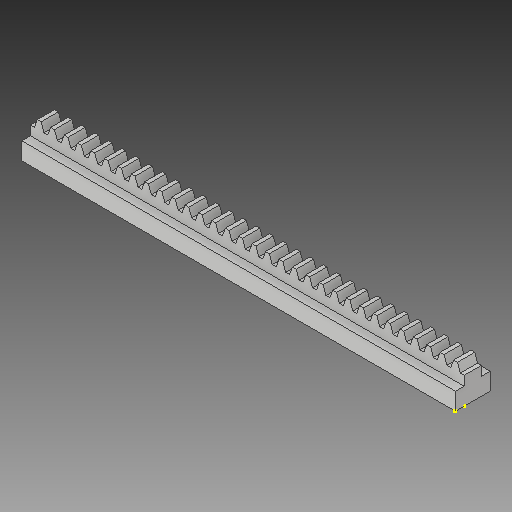
# Autodesk Inventor part: cremallera
Saved by Autodesk Inventor 2018.2 (Build 222227000, 227)
## iProperties
Created: 2016-05-04
Part Number: cremallera
Material: Genérico
Document SubType Name: Modeling
Designer: Usuario
Density: 1 g/cm^3
Appearance: Valor por defecto
Author: Usuario
Autodesk Inventor part; units mm, degrees
ref_plane "YZ Plane" through (0, 0, 0) normal (1, 0, 0) x (0, 1, 0)
ref_plane "XZ Plane" through (0, 0, 0) normal (0, 1, 0) x (-1, 0, 0)
ref_plane "XY Plane" through (0, 0, 0) normal (0, 0, 1) x (1, 0, 0)
sketch "Boceto1" plane through (0, 0, 0) normal (1, 0, 0) x (0, 1, 0)
  point P0 (0, 0)
extrude "Extrusión1" [suppressed]
sketch "Boceto2" plane through (0, 0, 0) normal (0, 0, 1) x (1, 0, 0)
  point P0 (0, 0)
sketch "Boceto3" plane through (0, 10, -5) normal (0, 0, 1) x (1, 0, 0)
  line L0 (227.2104, 2.6715) -> (229.8777, 10)
  line L1 (233.3764, 10) -> (236.0437, 2.6715)
  line L2 (214.787, 2.6715) -> (217.4544, 10)
  line L3 (220.953, 10) -> (223.6204, 2.6715)
  line L4 (202.3637, 2.6715) -> (205.031, 10)
  line L5 (208.5297, 10) -> (211.197, 2.6715)
  line L6 (189.9403, 2.6715) -> (192.6077, 10)
  line L7 (196.1063, 10) -> (198.7737, 2.6715)
  line L8 (177.517, 2.6715) -> (180.1843, 10)
  line L9 (183.683, 10) -> (186.3503, 2.6715)
  line L10 (165.0936, 2.6715) -> (167.761, 10)
  line L11 (171.2596, 10) -> (173.927, 2.6715)
  line L12 (152.6702, 2.6715) -> (155.3376, 10)
  line L13 (158.8362, 10) -> (161.5036, 2.6715)
  line L14 (140.2469, 2.6715) -> (142.9143, 10)
  line L15 (146.4129, 10) -> (149.0803, 2.6715)
  line L16 (127.8235, 2.6715) -> (130.4909, 10)
  line L17 (133.9895, 10) -> (136.6569, 2.6715)
  line L18 (115.4002, 2.6715) -> (118.0675, 10)
  line L19 (121.5662, 10) -> (124.2335, 2.6715)
  line L20 (102.9768, 2.6715) -> (105.6442, 10)
  line L21 (109.1428, 10) -> (111.8102, 2.6715)
  line L22 (90.5535, 2.6715) -> (93.2208, 10)
  line L23 (96.7195, 10) -> (99.3868, 2.6715)
  line L24 (78.1301, 2.6715) -> (80.7975, 10)
  line L25 (84.2961, 10) -> (86.9635, 2.6715)
  line L26 (65.7067, 2.6715) -> (68.3741, 10)
  line L27 (71.8728, 10) -> (74.5401, 2.6715)
  line L28 (53.2834, 2.6715) -> (55.9508, 10)
  line L29 (59.4494, 10) -> (62.1168, 2.6715)
  line L30 (40.86, 2.6715) -> (43.5274, 10)
  line L31 (47.0261, 10) -> (49.6934, 2.6715)
  line L32 (28.4367, 2.6715) -> (31.104, 10)
  line L33 (34.6027, 10) -> (37.2701, 2.6715)
  line L34 (16.0133, 2.6715) -> (18.6807, 10)
  line L35 (22.1793, 10) -> (24.8467, 2.6715)
  line L36 (3.59, 2.6715) -> (6.2573, 10)
  line L37 (9.756, 10) -> (12.4234, 2.6715)
  line L38 (239.6337, 2.6715) -> (242.3011, 10)
  line L39 (245.7997, 10) -> (248.4671, 2.6715)
  line L40 (248.4671, 2.6715) -> (250, 2.6715)
  line L41 (0, 0) -> (250, 0) projected
  line L42 (3.59, 2.6715) -> (0, 2.6715)
  line L43 (0, 0) -> (0, 10) projected
  line L44 (0, 2.6715) -> (0, 10)
  line L45 (0, 10) -> (6.2573, 10)
  line L46 (9.756, 10) -> (18.6807, 10)
  line L47 (12.4234, 2.6715) -> (16.0133, 2.6715)
  line L48 (236.0437, 2.6715) -> (239.6337, 2.6715)
  line L49 (223.6204, 2.6715) -> (227.2104, 2.6715)
  line L50 (211.197, 2.6715) -> (214.787, 2.6715)
  line L51 (198.7737, 2.6715) -> (202.3637, 2.6715)
  line L52 (186.3503, 2.6715) -> (189.9403, 2.6715)
  line L53 (173.927, 2.6715) -> (177.517, 2.6715)
  line L54 (161.5036, 2.6715) -> (165.0936, 2.6715)
  line L55 (149.0803, 2.6715) -> (152.6702, 2.6715)
  line L56 (136.6569, 2.6715) -> (140.2469, 2.6715)
  line L57 (124.2335, 2.6715) -> (127.8235, 2.6715)
  line L58 (111.8102, 2.6715) -> (115.4002, 2.6715)
  line L59 (99.3868, 2.6715) -> (102.9768, 2.6715)
  line L60 (86.9635, 2.6715) -> (90.5535, 2.6715)
  line L61 (74.5401, 2.6715) -> (78.1301, 2.6715)
  line L62 (62.1168, 2.6715) -> (65.7067, 2.6715)
  line L63 (49.6934, 2.6715) -> (53.2834, 2.6715)
  line L64 (24.8467, 2.6715) -> (28.4367, 2.6715)
  line L65 (37.2701, 2.6715) -> (40.86, 2.6715)
  line L66 (245.7997, 10) -> (250, 10)
  line L67 (233.3764, 10) -> (242.3011, 10)
  line L68 (220.953, 10) -> (229.8777, 10)
  line L69 (208.5297, 10) -> (217.4544, 10)
  line L70 (196.1063, 10) -> (205.031, 10)
  line L71 (183.683, 10) -> (192.6077, 10)
  line L72 (171.2596, 10) -> (180.1843, 10)
  line L73 (158.8362, 10) -> (167.761, 10)
  line L74 (146.4129, 10) -> (155.3376, 10)
  line L75 (133.9895, 10) -> (142.9143, 10)
  line L76 (121.5662, 10) -> (130.4909, 10)
  line L77 (109.1428, 10) -> (118.0675, 10)
  line L78 (96.7195, 10) -> (105.6442, 10)
  line L79 (84.2961, 10) -> (93.2208, 10)
  line L80 (59.4494, 10) -> (68.3741, 10)
  line L81 (71.8728, 10) -> (80.7975, 10)
  line L82 (47.0261, 10) -> (55.9508, 10)
  line L83 (34.6027, 10) -> (43.5274, 10)
  line L84 (22.1793, 10) -> (31.104, 10)
  line L85 (0, 10) -> (6.2573, 10)
  line L86 (9.756, 10) -> (18.6807, 10)
  line L87 (250, 10) -> (250, 2.6715)
  line L88 (250, 0) -> (250, 10) projected
  point P0 (0, -10)
  constraints: 172 end point, 19 parallel, 1 collinear, 1 horizontal, 1 point on line
extrude "Extrusión2" [suppressed]
sketch "Boceto4" plane through (0, 0, 0) normal (1, 0, 0) x (0, 1, 0)
  point P0 (0, 0)
extrude "Extrusión3" [suppressed]
sketch "Boceto5" plane through (0, 10, -5) normal (0, 0, 1) x (1, 0, 0)
  line L0 (-2.2374, 0.8668) -> (0, 0.865)
  line L1 (-17.723, 0.8787) -> (-13.2482, 0.8752)
  line L2 (-13.2482, 0.8752) -> (-9.9163, 10.0076)
  line L3 (-5.5553, 10.0043) -> (-2.2374, 0.8668)
  line L4 (-33.2086, 0.8905) -> (-28.7337, 0.8871)
  line L5 (-28.7337, 0.8871) -> (-25.4019, 10.0195)
  line L6 (-21.0409, 10.0162) -> (-17.723, 0.8787)
  line L7 (-48.6942, 0.9024) -> (-44.2194, 0.899)
  line L8 (-44.2194, 0.899) -> (-40.8875, 10.0314)
  line L9 (-36.5265, 10.028) -> (-33.2086, 0.8905)
  line L10 (-64.1798, 0.9143) -> (-59.7049, 0.9109)
  line L11 (-59.7049, 0.9109) -> (-56.3731, 10.0433)
  line L12 (-52.0121, 10.0399) -> (-48.6942, 0.9024)
  line L13 (-79.6654, 0.9262) -> (-75.1905, 0.9228)
  line L14 (-75.1905, 0.9228) -> (-71.8587, 10.0552)
  line L15 (-67.4976, 10.0518) -> (-64.1798, 0.9143)
  line L16 (-95.151, 0.9381) -> (-90.6761, 0.9347)
  line L17 (-90.6761, 0.9347) -> (-87.3443, 10.0671)
  line L18 (-82.9832, 10.0637) -> (-79.6654, 0.9262)
  line L19 (-110.6366, 0.95) -> (-106.1617, 0.9466)
  line L20 (-106.1617, 0.9466) -> (-102.8298, 10.0789)
  line L21 (-98.4688, 10.0756) -> (-95.151, 0.9381)
  line L22 (-121.6473, 0.9584) -> (-118.3155, 10.0908)
  line L23 (-113.9544, 10.0875) -> (-110.6366, 0.95)
  line L24 (-141.6008, 0.8651) -> (-137.1259, 0.8651)
  line L25 (-137.1259, 0.8651) -> (-133.8011, 10)
  line L26 (-129.4401, 10) -> (-126.1152, 0.8651)
  line L27 (-157.0864, 0.8651) -> (-152.6115, 0.8651)
  line L28 (-152.6115, 0.8651) -> (-149.2867, 10)
  line L29 (-144.9257, 10) -> (-141.6008, 0.8651)
  line L30 (-172.572, 0.8651) -> (-168.0971, 0.8651)
  line L31 (-168.0971, 0.8651) -> (-164.7723, 10)
  line L32 (-160.4113, 10) -> (-157.0864, 0.8651)
  line L33 (-188.0576, 0.8651) -> (-183.5827, 0.8651)
  line L34 (-183.5827, 0.8651) -> (-180.2579, 10)
  line L35 (-175.8969, 10) -> (-172.572, 0.8651)
  line L36 (-203.5432, 0.8651) -> (-199.0683, 0.8651)
  line L37 (-199.0683, 0.8651) -> (-195.7435, 10)
  line L38 (-191.3825, 10) -> (-188.0576, 0.8651)
  line L39 (-219.0288, 0.8651) -> (-214.5539, 0.8651)
  line L40 (-214.5539, 0.8651) -> (-211.2291, 10)
  line L41 (-206.868, 10) -> (-203.5432, 0.8651)
  line L42 (-234.5144, 0.8651) -> (-230.0395, 0.8651)
  line L43 (-230.0395, 0.8651) -> (-226.7147, 10)
  line L44 (-222.3537, 10) -> (-219.0288, 0.8651)
  line L45 (-250, 0.8651) -> (-245.5251, 0.8651)
  line L46 (-245.5251, 0.8651) -> (-242.2003, 10)
  line L47 (-237.8393, 10) -> (-234.5144, 0.8651)
  line L48 (0, 10) -> (-250, 10) projected
  line L49 (0, 0.865) -> (0, 10)
  line L50 (-250, 10) -> (-250, 0) projected
  line L51 (0, 10) -> (-5.5537, 10)
  line L52 (-9.9191, 10) -> (-21.035, 10)
  line L53 (-25.409, 10) -> (-36.5163, 10)
  line L54 (-40.8989, 10) -> (-51.9976, 10)
  line L55 (-56.3889, 10) -> (-67.4788, 10)
  line L56 (-71.8788, 10) -> (-82.9601, 10)
  line L57 (-87.3687, 10) -> (-98.4414, 10)
  line L58 (-102.8587, 10) -> (-113.9227, 10)
  line L59 (-118.3486, 10) -> (-129.4401, 10)
  line L60 (-133.8011, 10) -> (-144.9257, 10)
  line L61 (-149.2867, 10) -> (-160.4113, 10)
  line L62 (-164.7723, 10) -> (-175.8969, 10)
  line L63 (-180.2579, 10) -> (-191.3825, 10)
  line L64 (-195.7435, 10) -> (-206.868, 10)
  line L65 (-211.2291, 10) -> (-222.3537, 10)
  line L66 (-226.7147, 10) -> (-237.8393, 10)
  line L67 (-242.2003, 10) -> (-250, 10)
  line L68 (-250, 10) -> (-250, 0.8651)
  line L69 (-126.1152, 0.9584) -> (-121.6473, 0.9584)
  line L70 (-126.1265, 0.95) -> (-121.6516, 0.9466)
  line L71 (-121.6516, 0.9466) -> (-118.3198, 10.0789)
  line L72 (-129.4444, 10.0875) -> (-126.1265, 0.95)
  line L73 (-118.3486, 10) -> (-129.4126, 10)
  point P0 (0, -10)
  constraints: 144 end point, 19 horizontal, 18 point on line, 1 perpendicular, 1 vertical
extrude "Extrusión4" [suppressed]
sketch "Boceto6" plane through (-250, 10, -5) normal (0, 0, 1) x (1, 0, 0)
  point P0 (250, -10)
sketch "Boceto7" plane through (0, 0, 0) normal (1, 0, 0) x (0, 1, 0)
  line L0 (0, 0) -> (0, -20)
  line L1 (0, -20) -> (10, -20)
  line L2 (10, -20) -> (10, -15)
  line L3 (10, -15) -> (20, -15)
  line L4 (20, -15) -> (20, -5)
  line L5 (20, -5) -> (10, -5)
  line L6 (10, -5) -> (10, 0)
  line L7 (10, 0) -> (0, 0)
  constraints: 16 end point, 4 perpendicular, 2 point on line, 1 vertical
extrude "Extrusión5" add sketch "Boceto7" against normal blind 250
sketch "Boceto8" plane through (0, 10, -5) normal (0, 0, 1) x (1, 0, 0)
  line L0 (-110.6296, 5.4325) -> (-108.3922, 5.4325)
  line L1 (-108.3922, 5.4325) -> (-106.7297, 10)
  line L2 (-104.5492, 10) -> (-102.8868, 5.4325)
  line L3 (-118.3724, 5.4325) -> (-116.135, 5.4325)
  line L4 (-116.135, 5.4325) -> (-114.4725, 10)
  line L5 (-112.292, 10) -> (-110.6296, 5.4325)
  line L6 (-126.1152, 5.4325) -> (-123.8778, 5.4325)
  line L7 (-123.8778, 5.4325) -> (-122.2153, 10)
  line L8 (-120.0348, 10) -> (-118.3724, 5.4325)
  line L9 (-133.858, 5.4325) -> (-131.6206, 5.4325)
  line L10 (-131.6206, 5.4325) -> (-129.9581, 10)
  line L11 (-127.7776, 10) -> (-126.1152, 5.4325)
  line L12 (-141.6008, 5.4325) -> (-139.3634, 5.4325)
  line L13 (-139.3634, 5.4325) -> (-137.7009, 10)
  line L14 (-135.5204, 10) -> (-133.858, 5.4325)
  line L15 (-149.3436, 5.4325) -> (-147.1062, 5.4325)
  line L16 (-147.1062, 5.4325) -> (-145.4437, 10)
  line L17 (-143.2632, 10) -> (-141.6008, 5.4325)
  line L18 (-157.0864, 5.4325) -> (-154.849, 5.4325)
  line L19 (-154.849, 5.4325) -> (-153.1865, 10)
  line L20 (-151.006, 10) -> (-149.3436, 5.4325)
  line L21 (-164.8292, 5.4325) -> (-162.5918, 5.4325)
  line L22 (-162.5918, 5.4325) -> (-160.9293, 10)
  line L23 (-158.7488, 10) -> (-157.0864, 5.4325)
  line L24 (-172.572, 5.4325) -> (-170.3346, 5.4325)
  line L25 (-170.3346, 5.4325) -> (-168.6721, 10)
  line L26 (-166.4916, 10) -> (-164.8292, 5.4325)
  line L27 (-180.3148, 5.4325) -> (-178.0774, 5.4325)
  line L28 (-178.0774, 5.4325) -> (-176.4149, 10)
  line L29 (-174.2344, 10) -> (-172.572, 5.4325)
  line L30 (-188.0576, 5.4325) -> (-185.8202, 5.4325)
  line L31 (-185.8202, 5.4325) -> (-184.1577, 10)
  line L32 (-181.9772, 10) -> (-180.3148, 5.4325)
  line L33 (-195.8004, 5.4325) -> (-193.563, 5.4325)
  line L34 (-193.563, 5.4325) -> (-191.9005, 10)
  line L35 (-189.72, 10) -> (-188.0576, 5.4325)
  line L36 (-203.5432, 5.4325) -> (-201.3058, 5.4325)
  line L37 (-201.3058, 5.4325) -> (-199.6433, 10)
  line L38 (-197.4628, 10) -> (-195.8004, 5.4325)
  line L39 (-211.286, 5.4325) -> (-209.0486, 5.4325)
  line L40 (-209.0486, 5.4325) -> (-207.3861, 10)
  line L41 (-205.2056, 10) -> (-203.5432, 5.4325)
  line L42 (-219.0288, 5.4325) -> (-216.7914, 5.4325)
  line L43 (-216.7914, 5.4325) -> (-215.1289, 10)
  line L44 (-212.9484, 10) -> (-211.286, 5.4325)
  line L45 (-226.7716, 5.4325) -> (-224.5342, 5.4325)
  line L46 (-224.5342, 5.4325) -> (-222.8717, 10)
  line L47 (-220.6912, 10) -> (-219.0288, 5.4325)
  line L48 (-234.5144, 5.4325) -> (-232.277, 5.4325)
  line L49 (-232.277, 5.4325) -> (-230.6145, 10)
  line L50 (-228.434, 10) -> (-226.7716, 5.4325)
  line L51 (-242.2572, 5.4325) -> (-240.0198, 5.4325)
  line L52 (-240.0198, 5.4325) -> (-238.3573, 10)
  line L53 (-236.1768, 10) -> (-234.5144, 5.4325)
  line L54 (-250, 5.4325) -> (-247.7626, 5.4325)
  line L55 (-247.7626, 5.4325) -> (-246.1001, 10)
  line L56 (-243.9196, 10) -> (-242.2572, 5.4325)
  line L57 (-250, 5.4325) -> (-250, 10)
  line L58 (-250, -10) -> (-250, 0) projected
  line L59 (-2.2304, 5.4325) -> (0, 5.4325)
  line L60 (-9.9732, 5.4325) -> (-7.7358, 5.4325)
  line L61 (-7.7358, 5.4325) -> (-6.0734, 10)
  line L62 (-3.8928, 10) -> (-2.2304, 5.4325)
  line L63 (-17.716, 5.4325) -> (-15.4786, 5.4325)
  line L64 (-15.4786, 5.4325) -> (-13.8162, 10)
  line L65 (-11.6356, 10) -> (-9.9732, 5.4325)
  line L66 (-25.4588, 5.4325) -> (-23.2214, 5.4325)
  line L67 (-23.2214, 5.4325) -> (-21.559, 10)
  line L68 (-19.3784, 10) -> (-17.716, 5.4325)
  line L69 (-33.2016, 5.4325) -> (-30.9642, 5.4325)
  line L70 (-30.9642, 5.4325) -> (-29.3017, 10)
  line L71 (-27.1212, 10) -> (-25.4588, 5.4325)
  line L72 (-40.9444, 5.4325) -> (-38.707, 5.4325)
  line L73 (-38.707, 5.4325) -> (-37.0446, 10)
  line L74 (-34.864, 10) -> (-33.2016, 5.4325)
  line L75 (-48.6872, 5.4325) -> (-46.4498, 5.4325)
  line L76 (-46.4498, 5.4325) -> (-44.7874, 10)
  line L77 (-42.6068, 10) -> (-40.9444, 5.4325)
  line L78 (-56.43, 5.4325) -> (-54.1926, 5.4325)
  line L79 (-54.1926, 5.4325) -> (-52.5302, 10)
  line L80 (-50.3496, 10) -> (-48.6872, 5.4325)
  line L81 (-64.1728, 5.4325) -> (-61.9354, 5.4325)
  line L82 (-61.9354, 5.4325) -> (-60.273, 10)
  line L83 (-58.0924, 10) -> (-56.43, 5.4325)
  line L84 (-71.9156, 5.4325) -> (-69.6782, 5.4325)
  line L85 (-69.6782, 5.4325) -> (-68.0157, 10)
  line L86 (-65.8352, 10) -> (-64.1728, 5.4325)
  line L87 (-79.6584, 5.4325) -> (-77.421, 5.4325)
  line L88 (-77.421, 5.4325) -> (-75.7585, 10)
  line L89 (-73.578, 10) -> (-71.9156, 5.4325)
  line L90 (-87.4012, 5.4325) -> (-85.1638, 5.4325)
  line L91 (-85.1638, 5.4325) -> (-83.5014, 10)
  line L92 (-81.3208, 10) -> (-79.6584, 5.4325)
  line L93 (-95.144, 5.4325) -> (-92.9066, 5.4325)
  line L94 (-92.9066, 5.4325) -> (-91.2442, 10)
  line L95 (-89.0636, 10) -> (-87.4012, 5.4325)
  line L96 (-102.8868, 5.4325) -> (-100.6494, 5.4325)
  line L97 (-100.6494, 5.4325) -> (-98.987, 10)
  line L98 (-96.8064, 10) -> (-95.144, 5.4325)
  line L99 (-3.8928, 10) -> (0.007, 10)
  line L100 (-11.6356, 10) -> (-6.0734, 10)
  line L101 (-19.3784, 10) -> (-13.8162, 10)
  line L102 (-27.1212, 10) -> (-21.559, 10)
  line L103 (-34.864, 10) -> (-29.3017, 10)
  line L104 (-42.6068, 10) -> (-37.0446, 10)
  line L105 (-50.3496, 10) -> (-44.7874, 10)
  line L106 (-58.0924, 10) -> (-52.5302, 10)
  line L107 (-81.3208, 10) -> (-75.7585, 10)
  line L108 (-89.0636, 10) -> (-83.5014, 10)
  line L109 (-96.8064, 10) -> (-91.2442, 10)
  line L110 (-104.5492, 10) -> (-98.987, 10)
  line L111 (-112.292, 10) -> (-106.7297, 10)
  line L112 (-120.0348, 10) -> (-114.4725, 10)
  line L113 (-127.7776, 10) -> (-122.2153, 10)
  line L114 (-135.5204, 10) -> (-129.9581, 10)
  line L115 (-143.2632, 10) -> (-137.7009, 10)
  line L116 (-151.006, 10) -> (-145.4437, 10)
  line L117 (-158.7488, 10) -> (-153.1865, 10)
  line L118 (-166.4916, 10) -> (-160.9293, 10)
  line L119 (-174.2344, 10) -> (-168.6721, 10)
  line L120 (-181.9772, 10) -> (-176.4149, 10)
  line L121 (-189.72, 10) -> (-184.1577, 10)
  line L122 (-197.4628, 10) -> (-191.9005, 10)
  line L123 (-205.2056, 10) -> (-199.6433, 10)
  line L124 (-212.9484, 10) -> (-207.3861, 10)
  line L125 (-220.6912, 10) -> (-215.1289, 10)
  line L126 (-228.434, 10) -> (-222.8717, 10)
  line L127 (-236.1768, 10) -> (-230.6145, 10)
  line L128 (-250, 10) -> (-246.1001, 10)
  line L129 (-243.9196, 10) -> (-238.3573, 10)
  line L130 (-73.578, 10) -> (-68.0157, 10)
  line L131 (-65.8352, 10) -> (-60.273, 10)
  line L132 (-100.6494, 5.4325) -> (-98.987, 10)
  line L133 (-102.8868, 5.4325) -> (-100.6494, 5.4325)
  line L134 (-104.5492, 10) -> (-102.8868, 5.4325)
  line L135 (-104.5492, 10) -> (-98.987, 10)
  line L136 (-250, 10) -> (-246.1001, 10)
  line L137 (-246.1001, 10) -> (-247.7626, 5.4325)
  line L138 (-250, 5.4325) -> (-250, 10)
  line L139 (0, 10) -> (-250, 10) projected
  line L140 (0, 10) -> (0, 5.4325)
  line L141 (0, 10) -> (0, 0) projected
  line L142 (0, 10) -> (-3.8928, 10)
  line L143 (-2.2304, 5.4325) -> (0, 5.4325)
  point P0 (0, -10)
  constraints: 282 end point, 36 horizontal, 1 collinear, 1 parallel, 1 perpendicular, 1 vertical
extrude "Extrusión6" cut sketch "Boceto8" against normal blind 10
